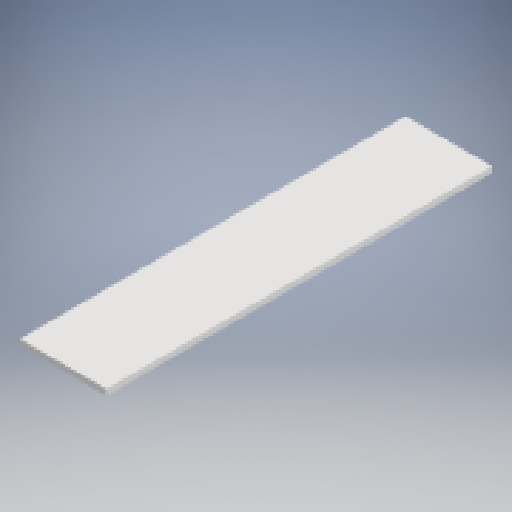
# Autodesk Inventor part: SIDE SH
Saved by Autodesk Inventor 2025.2 (Build 292293000, 293)
## iProperties
Created: 2025-01-29
Part Number: SIDE SH
Material: Generic
Document SubType Name: Modeling
Designer: Anna
Density: 1 g/cm^3
Appearance: Default
Author: Anna
Autodesk Inventor part; units mm, degrees
ref_plane "YZ Plane" through (0, 0, 0) normal (1, 0, 0) x (0, 1, 0)
ref_plane "XZ Plane" through (0, 0, 0) normal (0, 1, 0) x (-1, 0, 0)
ref_plane "XY Plane" through (0, 0, 0) normal (0, 0, 1) x (1, 0, 0)
sketch "Sketch1" plane through (0, 0, 0) normal (1, 0, 0) x (0, 1, 0)
  line L0 (0, 622.3) -> (0, -622.3)
  line L1 (0, 622.3) -> (19.05, 622.3)
  line L2 (19.05, 622.3) -> (19.05, -622.3)
  line L3 (19.05, -622.3) -> (0, -622.3)
  point P0 (0, 0)
  dimension "d0" = 1244.6
  dimension "d1" = 19.05
  constraints: 8 end point, 2 perpendicular, 1 horizontal, 1 midpoint, 1 vertical
  measures "d0" distance of L0.start L0.end
  measures "d1" distance of L0.start L1.end
extrude "Extrusion1" add sketch "Sketch1" along normal blind 279.4
body "Solid1"
